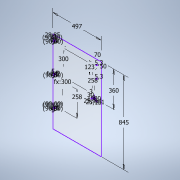
# Autodesk Inventor part: Plexiglas_Einfassung_550x710mm
Saved by Autodesk Inventor 2022 (Build 260153000, 153)
## iProperties
Created: 2020-11-17
Part Number: Plexiglas_Einfassung_550x710mm
Material: Polycarbonate, Clear
Document SubType Name: Modeling
Designer: Alexander Fritzsche
Density: 1.2 g/cm^3
Appearance: Polycarbonate - Clear
Author: Alexander Fritzsche
Autodesk Inventor part; units mm, degrees
ref_plane "YZ Plane" through (0, 0, 0) normal (1, 0, 0) x (0, 1, 0)
ref_plane "XZ Plane" through (0, 0, 0) normal (0, 1, 0) x (-1, 0, 0)
ref_plane "XY Plane" through (0, 0, 0) normal (0, 0, 1) x (1, 0, 0)
sketch "Sketch1" plane through (0, 0, 0) normal (0, 0, 1) x (1, 0, 0)
  line L0 (17.0037, 144.1779) -> (514.0037, 144.1779)
  line L1 (514.0037, 144.1779) -> (514.0037, 949.1779)
  line L2 (514.0037, 949.1779) -> (17.0037, 949.1779)
  circle A0 centre (469.9509, 776.1779) radius 2.65
  circle A1 centre (469.9509, 899.1779) radius 2.65
  circle A2 centre (444.0037, 589.1779) radius 15
  circle A3 centre (444.0037, 619.1779) radius 1.5
  circle A4 centre (418.023, 574.1779) radius 1.5
  circle A5 centre (469.9845, 574.1779) radius 1.5
  line L3 (444.0037, 589.1779) -> (444.0037, 619.1779) construction
  line L4 (444.0037, 589.1779) -> (444.0037, 619.1779) construction
  line L5 (444.0037, 589.1779) -> (444.0037, 619.1779) construction
  line L6 (444.0037, 589.1779) -> (444.0037, 619.1779) construction
  line L7 (17.0037, 949.1779) -> (17.0037, 920.3279)
  line L8 (17.0037, 920.3279) -> (22.0037, 920.3279)
  line L9 (22.0037, 920.3279) -> (22.0037, 878.3279)
  line L10 (22.0037, 878.3279) -> (17.0037, 878.3279)
  line L11 (17.0037, 878.3279) -> (17.0037, 620.3279)
  line L12 (17.0037, 620.3279) -> (22.0037, 620.3279)
  line L13 (22.0037, 620.3279) -> (22.0037, 578.3279)
  line L14 (22.0037, 578.3279) -> (17.0037, 578.3279)
  line L15 (17.0037, 578.3279) -> (17.0037, 320.3279)
  line L16 (17.0037, 320.3279) -> (22.0037, 320.3279)
  line L17 (22.0037, 320.3279) -> (22.0037, 278.3279)
  line L18 (22.0037, 278.3279) -> (17.0037, 278.3279)
  line L19 (17.0037, 144.1779) -> (17.0037, 278.3279)
  line L20 (35.5037, 901.6779) -> (38.0037, 901.6779)
  line L21 (35.5037, 896.6779) -> (38.0037, 896.6779)
  arc A6 (35.5037, 901.6779) -> (35.5037, 896.6779) centre (35.5037, 899.1779) ccw
  arc A7 (38.0037, 896.6779) -> (38.0037, 901.6779) centre (38.0037, 899.1779) ccw
  line L22 (35.5037, 601.6779) -> (38.0037, 601.6779)
  line L23 (35.5037, 596.6779) -> (38.0037, 596.6779)
  line L24 (35.5037, 301.6779) -> (38.0037, 301.6779)
  line L25 (35.5037, 296.6779) -> (38.0037, 296.6779)
  arc A8 (35.5037, 301.6779) -> (35.5037, 296.6779) centre (35.5037, 299.1779) ccw
  arc A9 (38.0037, 296.6779) -> (38.0037, 301.6779) centre (38.0037, 299.1779) ccw
  arc A10 (35.5037, 601.6779) -> (35.5037, 596.6779) centre (35.5037, 599.1779) ccw
  arc A11 (38.0037, 596.6779) -> (38.0037, 601.6779) centre (38.0037, 599.1779) ccw
  dimension "d72" = 497
  dimension "d73" = 805
  dimension "d85" = 50
  dimension "d133" = 5.3
  dimension "d134" = 5.3
  dimension "d135" = 123
  dimension "d168" = 50
  dimension "d218" = 30
  dimension "d219" = 70
  dimension "d221" = 3
  dimension "d222" = 3
  dimension "d223" = 3
  dimension "d224" = 30
  dimension "d228" = 15
  dimension "d230" = 15
  dimension "d231" = 25.9808
  dimension "d232" = 25.9808
  dimension "d233" = 360
  dimension "d248" = 300
  dimension "d249" = 300
  dimension "d250" = 28.85
  dimension "d251" = 5
  dimension "d252" = 42
  dimension "d253" = 90
  dimension "d254" = 5
  dimension "d255" = 90
  dimension "d256" = 21
  dimension "d257" = 5
  dimension "d258" = 42
  dimension "d259" = 5
  dimension "d260" = 90
  dimension "d261" = 5
  dimension "d262" = 90
  dimension "d263" = 42
  dimension "d264" = 90
  dimension "d265" = 5
  dimension "d266" = 90
  dimension "d268" = 258
  dimension "d269" = 258
  dimension "d270" = 2.5
  dimension "d271" = 5
  dimension "d272" = 7.5
  dimension "d273" = 5
  dimension "d274" = 7.5
  dimension "d275" = 2.5
  dimension "d276" = 7.5
  dimension "d277" = 2.5
  dimension "d278" = 5
  constraints: 52 end point, 12 centre point, 12 point on circle, 10 perpendicular, 4 tangent, 4 vertical alignment, 3 coincident, 3 horizontal, 3 parallel, 3 vertical, 1 point on line
  measures "d72" distance of L2.end L1.end
  measures "d73" distance of L1.end L0.end
  measures "d85" distance from line of L2 A7.centre
  measures "d133" diameter of A0
  measures "d134" diameter of A1
  measures "d135" distance of A1.centre A0.centre
  measures "d168" distance from line of L2 A1.centre
  measures "d218" diameter of A2
  measures "d219" distance from line of L1 A2.centre
  measures "d221" diameter of A3
  measures "d222" diameter of A4
  measures "d223" diameter of A5
  measures "d224" distance of A2.centre L3.end
  measures "d228" vertical distance of A4.centre A2.centre
  measures "d230" vertical distance of A5.centre A2.centre
  measures "d231" horizontal distance of A4.centre A2.centre
  measures "d232" horizontal distance of A5.centre A2.centre
  measures "d233" distance from line of L2 A2.centre
  measures "d248" distance of A11.centre A7.centre
  measures "d249" distance of A11.centre A9.centre
  measures "d250" distance of L2.end L7.end
  measures "d251" distance of L7.end L8.end
  measures "d252" distance of L8.end L9.end
  measures "d253" angle of L8 L9
  measures "d254" distance of L9.end L10.end
  measures "d255" angle of L9 L10
  measures "d256" distance from line of L7 A7.centre
  measures "d257" distance of L11.end L12.end
  measures "d258" distance of L12.end L13.end
  measures "d259" distance of L13.end L14.end
  measures "d260" angle of L13 L14
  measures "d261" distance of L15.end L16.end
  measures "d262" angle of L16 L15
  measures "d263" distance of L16.end L17.end
  measures "d264" angle of L16 L17
  measures "d265" distance of L17.end L18.end
  measures "d266" angle of L17 L18
  measures "d268" distance of L10.end L11.end
  measures "d269" distance of L14.end L15.end
  measures "d270" distance of A7.centre A6.centre
  measures "d271" distance between parallel lines of L21 L20
  measures "d273" distance between parallel lines of L22 L23
  measures "d275" distance of A11.centre A10.centre
  measures "d277" distance of A9.centre A8.centre
  measures "d278" distance between parallel lines of L25 L24
extrude "Extrusion2" add sketch "Sketch1" along normal blind 3 contours L19 L18 L17 L16 L15 L14 L13 L12 L11 L10 L9 L8 L7 L2 L1 L0 | A0 | A1 | A2 | A3 | A4 | A5 | L20 A7 L21 A6 | L22 A11 L23 A10 | L24 A9 L25 A8
hole "Hole7" at (38.0037, 899.1779, 0) direction (0, 0, 1) diameter 5 end through all
hole "Hole8" at (38.0037, 599.1779, 0) direction (0, 0, 1) diameter 5 end through all
hole "Hole9" at (38.0037, 299.1779, 0) direction (0, 0, 1) diameter 5 end through all
hole "Hole13" at (469.9509, 776.1779, 0) direction (0, 0, 1) diameter 5.3 end through all
hole "Hole14" at (469.9509, 899.1779, 0) direction (0, 0, 1) diameter 5.3 end through all
extrude "Extrusion7" cut sketch "Sketch1" along normal blind 10 contours A2
extrude "Extrusion8" cut sketch "Sketch1" along normal blind 10 contours A3
extrude "Extrusion9" cut sketch "Sketch1" along normal blind 10 contours A4
extrude "Extrusion10" cut sketch "Sketch1" along normal blind 10 contours A5
equation "\"d91\" = d81"
equation "\"d98\" = d81"
equation "\"d105\" = d81"
equation "\"d137\" = d133"
equation "\"d144\" = d133"
equation "\"d81\" = 5"
body "Solid2"
